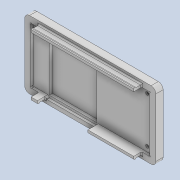
# Autodesk Inventor part: scatola_v2_sotto
Saved by Autodesk Inventor 2022 (Build 260153000, 153)
## iProperties
Created: 2025-09-23
Part Number: scatola_v2_sotto
Material: Generic
Document SubType Name: Modeling
Designer: 1234
Density: 1 g/cm^3
Appearance: Default
Author: 1234
Autodesk Inventor part; units mm, degrees
ref_plane "YZ Plane" through (0, 0, 0) normal (1, 0, 0) x (0, 1, 0)
sketch "Sketch1" plane through (0, 0, 0) normal (0, 0, 1) x (1, 0, 0)
  line L0 (0, 0) -> (-75, 0)
  line L1 (-75, 0) -> (-75, 35)
  line L2 (-75, 35) -> (0, 35)
  line L3 (0, 35) -> (0, 0)
  line L4 (4, -4) -> (-79, -4)
  line L5 (-79, -4) -> (-79, 39)
  line L6 (-79, 39) -> (4, 39)
  line L7 (4, 39) -> (4, -4)
  line L8 (-37.5, 39) -> (-37.5, 56.2273) construction
  line L9 (-79, 17.5) -> (-92.6498, 17.5) construction
  line L10 (-65, 0) -> (-65, 35)
  line L11 (-35, 0) -> (-35, 35)
  circle A0 centre (-3, 32) radius 1
  circle A1 centre (-3, 3) radius 1
  line L12 (-3, 3) -> (-3, 32) construction
  line L13 (-3, 17.5) -> (-10.1857, 17.5) construction
  circle A2 centre (-75, 35) radius 0.5
  circle A3 centre (0, 35) radius 0.5
  circle A4 centre (-75, 0) radius 0.5
  circle A5 centre (0, 0) radius 0.5
  line L14 (-75.2, 35.2) -> (-75.2, -0.2)
  line L15 (-75.2, -0.2) -> (0.2, -0.2)
  line L16 (0.2, -0.2) -> (0.2, 35.2)
  line L17 (0.2, 35.2) -> (-75.2, 35.2)
  line L18 (-65, 0) -> (-65, -1.5)
  line L19 (-65, -1.5) -> (-35, -1.5)
  line L20 (-35, -1.5) -> (-35, 0)
  point P0 (-0.5, 35)
  point P1 (0, 34.5)
  point P2 (0, 0.5)
  point P3 (-0.5, 0)
  point P4 (-75, 0.5)
  point P5 (-74.5, 0)
  point P6 (-74.5, 35)
  point P7 (-75, 34.5)
  point P8 (0.2, 0.4583)
  point P9 (0.2, 34.5417)
  point P10 (-0.4583, 35.2)
  point P11 (-74.5417, 35.2)
  point P12 (-74.5417, -0.2)
  point P13 (-0.4583, -0.2)
  point P14 (-75.2, 34.5417)
  point P15 (-75.2, 0.4583)
  point P16 (-35, -0.2)
  point P17 (-65, -0.2)
  dimension "d0" = 75
  dimension "d1" = 35
  dimension "d2" = 4
  dimension "d8" = 10
  dimension "d9" = 40
  dimension "d10" = 2
  dimension "d11" = 2
  dimension "d12" = 29
  dimension "d13" = 3
  dimension "d18" = 1
  dimension "d21" = 75
  dimension "d24" = 35
  dimension "d32" = 0.2
  dimension "d33" = 1.5
  constraints: 42 end point, 9 perpendicular, 6 centre point, 6 parallel, 4 point on line, 3 horizontal, 3 midpoint, 3 vertical, 1 coincident, 1 collinear, 12 other
  measures "d0" distance of L1.end L2.end
  measures "d1" distance of L0.end L1.end
  measures "d2" distance between parallel lines of L3 L7
  measures "d8" distance between parallel lines of L1 L10
  measures "d9" distance between parallel lines of L1 L11
  measures "d10" diameter of A1
  measures "d11" diameter of A0
  measures "d12" distance of L12.start L12.end
  measures "d13" distance between parallel lines of L3 L12
  measures "d18" diameter of A2
  measures "d21" distance of A2.centre A3.centre
  measures "d24" distance of A2.centre A4.centre
  measures "d32" distance between parallel lines of L1 L14
  measures "d33" distance between parallel lines of L0 L19
extrude "Extrusion1" add sketch "Sketch1" along normal blind 4.6 contours L20 L15 L18 L0 | L11 L2 A3 L3 A5 L0 | L0 L10 L2 L11 | L0 A5 L15 L20 | L18 L15 A4 L0 | L0 A4 L1 A2 L2 L10 | A5 L3 L0 | L0 L3 A5 L16 L15 | L2 A2 L17 A3 | L20 L19 L18 L15 | A4 L15 L14 L1 L0 | L0 L1 A4 | L3 A3 L16 A5 | L15 L16 A5 | A3 L17 L16 L3 L2 | L2 L3 A3 | A4 L14 A2 L1 | A4 L14 L15 | A2 L1 L2 | L2 L1 A2 L14 L17 | A3 L16 L17 | L17 L14 A2 | L4 L5 L6 L7 | A0 | A1
extrude "Extrusion2" cut sketch "Sketch1" against normal blind 1.6 from surface at 4.6 contours L20 L15 L18 L0 | L11 L2 A3 L3 A5 L0 | L0 L10 L2 L11 | L0 A5 L15 L20 | L18 L15 A4 L0 | L0 A4 L1 A2 L2 L10 | A5 L3 L0 | L0 L3 A5 L16 L15 | L2 A2 L17 A3 | L20 L19 L18 L15 | A4 L15 L14 L1 L0 | L0 L1 A4 | L3 A3 L16 A5 | L15 L16 A5 | A3 L17 L16 L3 L2 | L2 L3 A3 | A4 L14 A2 L1 | A4 L14 L15 | A2 L1 L2 | L2 L1 A2 L14 L17 | A3 L16 L17 | L17 L14 A2 | A0 | A1
extrude "Extrusion3" cut sketch "Sketch1" against normal blind 2 from surface at 3 contours L0 L10 L2 L11
extrude "Extrusion4" cut sketch "Sketch1" against normal blind 3 from surface at 3 contours A0 | A1
chamfer "Chamfer2" distance 1 angle 45 2 edges at (-65, -0.2, 3.8) (-35, -0.2, 3.8)
fillet "Fillet1" radius 3 4 edges at (4, 39, 2.3) (-79, 39, 2.3) (-79, -4, 2.3) (4, -4, 2.3)
ref_plane "Work Plane1" through (-37.5, -1, 0) normal (1, 0, 0) x (0, 0, -1)
sketch "Sketch2" plane through (-37.5, -1, 0) normal (1, 0, 0) x (0, 0, -1)
  line L0 (-1, 1) -> (-3, 1) projected
  line L1 (-3, 1) -> (-4.6, 1)
  line L2 (-4.6, -3) -> (-4.6, 0) projected
  line L3 (-4.6, -0.8) -> (-4.6, 0.8)
  line L4 (-9.6, 0.8) -> (-9.6, -0.8)
  line L5 (-9.6, -0.8) -> (-4.6, -0.8)
  line L6 (-9.6, -0.8) -> (-9.6, -1.25)
  line L7 (-9.6, -1.25) -> (-8.6, -1.25)
  line L8 (-8.6, -1.25) -> (-8.15, -0.8)
  line L9 (-9.6, -0.8) -> (-9.15, -1.25)
  line L10 (-9.6, 0.8) -> (-4.6, 0.8)
  line L11 (-3, 0.8) -> (-4.6, 0.8) projected
  point P0 (0, 1)
  point P1 (-4.6, 1)
  point P2 (-4.6, -0.2)
  dimension "d41" = 1.6
  dimension "d42" = 0.45
  dimension "d45" = 45
  dimension "d46" = 45
  dimension "d47" = 1
  dimension "d51" = 5
  constraints: 16 end point, 4 perpendicular, 3 point on line, 2 vertical, 1 collinear, 3 other
  measures "d41" distance of L4.start L4.end
  measures "d42" distance of L4.end L6.end
  measures "d45" angle of L5 L8
  measures "d46" angle of L9 L5
  measures "d47" distance of L6.end L7.end
  measures "d51" distance of L4.start L10.end
ref_plane "Work Plane2" through (-67.5, -1, 0) normal (1, 0, 0) x (0, 0, -1)
extrude "Extrusion5" add sketch "Sketch2" against normal blind 32.5 and the other way blind 3.5 contours L5 L4 L10 L3 L2 | L8 L7 L9 L5
ref_plane "Work Plane3" through (-76, 17.5, 0) normal (0, 1, 0) x (1, 0, 0)
mirror "Mirror1" about plane through (-37.5, -1, 0) normal (1, 0, 0) of "Extrusion5"
fillet "Fillet4" radius 0.8 3 edges at (-37.5, -1.8, 4.6) (-5, -1, 4.6) (-70, -1, 4.6)
mirror "Mirror2" about plane through (-76, 17.5, 0) normal (0, 1, 0) of "Extrusion5", "Mirror1", "Fillet4"
sketch "Sketch7" plane through (0, 0, 4.6) normal (0, 0, 1) x (1, 0, 0)
  line L0 (-66, -0.2) -> (-66, -4)
  line L1 (-66, -4) -> (-34, -4)
  line L2 (-76, -4) -> (1, -4) projected
  line L3 (-34, -0.2) -> (-35, -1.2) projected
  line L4 (-34, -0.2) -> (-34, -4)
  line L5 (-66, -0.2) -> (-34, -0.2)
  point P0 (0, 0)
  constraints: 8 end point, 2 point on line, 2 vertical, 1 horizontal
extrude "Extrusion10" cut sketch "Sketch7" along normal through all
fillet "Fillet5" radius 0.8 2 edges at (-66, -1.4, 4.6) (-34, -1.4, 4.6)
sketch "Sketch3" plane through (4, -1, 4.6) normal (1, 0, 0) x (0, 0, -1)
  line L0 (-8.3163, -11.6343) -> (11.7066, -11.6343)
  line L1 (11.7066, -11.6343) -> (11.7066, 46.4717)
  line L2 (11.7066, 46.4717) -> (-8.3163, 46.4717)
  line L3 (-8.3163, 46.4717) -> (-8.3163, -11.6343)
  point P0 (4.6, 1)
  constraints: 8 end point, 2 parallel, 1 horizontal, 1 perpendicular
sketch "Sketch4" plane through (-74.5417, 35.2, 3) normal (0, 0, 1) x (1, 0, 0)
  line L0 (-6.3289, -41.6688) -> (13.4056, -41.6688)
  line L1 (13.4056, -41.6688) -> (13.4056, 7.8526)
  line L2 (13.4056, 7.8526) -> (-6.3289, 7.8526)
  line L3 (-6.3289, 7.8526) -> (-6.3289, -41.6688)
  point P0 (74.5417, -35.2)
  constraints: 8 end point, 2 parallel, 1 horizontal, 1 perpendicular
sketch "Sketch5" plane through (-74.5417, 35.2, 4.6) normal (0, 0, -1) x (-1, 0, 0)
  line L0 (-3.0733, -37.6) -> (-8.5102, -37.6) projected
  line L1 (-3.6554, 1.6179) -> (-3.0733, 2.2) projected
  line L2 (-8.5102, -37.6) -> (-3.0733, -37.6)
  line L3 (-3.0733, -37.6) -> (-3.0733, 2.2)
  line L4 (-3.0733, 2.2) -> (-8.5102, 2.2)
  line L5 (-8.5102, 2.2) -> (-8.5102, -37.6)
  point P0 (-74.5417, -35.2)
  constraints: 8 end point, 2 parallel, 1 horizontal, 1 perpendicular
sketch "Sketch6" plane through (-74.5417, 35.2, 4.6) normal (0, 0, 1) x (1, 0, 0)
  line L0 (3.0733, -37.6) -> (3.0733, 2.2) projected
  line L1 (8.5102, 2.2) -> (8.5102, -37.6) projected
  line L2 (3.0733, 0.0729) -> (8.5102, 0.0729)
  line L3 (8.5102, 0.0729) -> (8.5102, -35.4359)
  line L4 (8.5102, -35.4359) -> (3.0733, -35.4359)
  line L5 (3.0733, -35.4359) -> (3.0733, 0.0729)
  point P0 (74.5417, -35.2)
  point P1 (3.0733, -35.4359)
  constraints: 8 end point, 2 parallel, 2 point on line, 1 horizontal, 1 perpendicular
equation "\"d11\" = d10"
equation "\"d21\" = d0"
equation "\"d24\" = d1"
body "Solid1"
